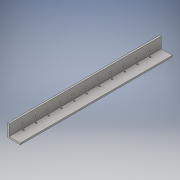
# Autodesk Inventor part: Fer Angle
Saved by Autodesk Inventor 2016 (Build 200138000, 138)
## iProperties
Created: 2016-02-02
Part Number: Fer Angle
Material: Generic
Document SubType Name: Modeling
Designer: ares-b02
Density: 1 g/cm^3
Appearance: Default
Author: ares-b02
Autodesk Inventor part; units mm, degrees
ref_plane "YZ Plane" through (0, 0, 0) normal (1, 0, 0) x (0, 1, 0)
ref_plane "XZ Plane" through (0, 0, 0) normal (0, 1, 0) x (-1, 0, 0)
ref_plane "XY Plane" through (0, 0, 0) normal (0, 0, 1) x (1, 0, 0)
sketch "Sketch1" plane through (0, 0, 0) normal (0, 0, 1) x (1, 0, 0)
  line L0 (0, 25.4) -> (0, 0)
  line L1 (0, 0) -> (25.4, 0)
  line L2 (25.4, 0) -> (25.4, 3.175)
  line L3 (25.4, 3.175) -> (3.175, 3.175)
  line L4 (3.175, 3.175) -> (3.175, 25.4)
  line L5 (3.175, 25.4) -> (0, 25.4)
  dimension "d11" = 25.4
  dimension "d12" = 25.4
  dimension "d13" = 3.175
  dimension "d14" = 3.175
  constraints: 12 end point, 4 perpendicular, 1 parallel, 1 vertical
  measures "d11" distance of L0.end L1.end
  measures "d12" distance of L0.start L0.end
  measures "d13" distance of L4.end L0.start
  measures "d14" distance of L1.end L2.end
extrude "Extrusion1" add sketch "Sketch1" along normal blind 304.8
hole "Hole1" at (6.35, 0, 25.4) direction (0, 1, 0) diameter 3.175 end through all
hole "Hole2" at (0, 12.7, 25.4) direction (1, 0, 0) diameter 3.175 end through all
pattern_linear "Rectangular Pattern1" count 11 spacing 25.4 along (0, 0, 1) of "Hole1"
pattern_linear "Rectangular Pattern2" count 11 spacing 25.4 along (0, 0, 1) of "Hole2"
body "Solid1"
